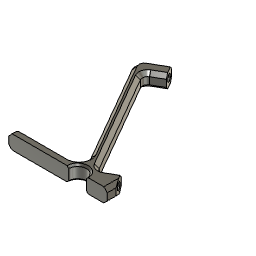
CYD Stand Leg Portrait (Autodesk Fusion 360 design; units mm, degrees)
Autodesk Fusion 360 part; units mm, degrees
sketch "Sketch1" plane through (0, 0, 0) normal (0, 0, 1) x (1, 0, 0)
  line L0 (0, 0) -> (55.9904, 0)
  line L1 (55.9904, 0) -> (55.9904, 5)
  line L2 (30.0096, 5) -> (3, 5)
  line L3 (0, 5) -> (0, 0)
  line L4 (34.3397, 12.5) -> (2.5, 67.6481)
  line L5 (41.5566, 0) -> (125.219, 0) construction
  line L6 (9.8301, 64.9519) -> (41.8301, 9.5263)
  line L7 (4.3301, 74.4782) -> (12.9904, 79.4782)
  line L8 (12.9904, 79.4782) -> (16.9904, 72.55)
  line L9 (16.9904, 72.55) -> (10.9282, 69.05)
  line L10 (14.9904, 76.0141) -> (36.6637, 88.5272) construction
  line L11 (0, 2) -> (0, 0) construction
  line L12 (55.9904, 5) -> (51.9904, 11.9282)
  line L13 (51.9904, 11.9282) -> (45.9282, 8.4282)
  arc A0 (4.3301, 74.4782) -> (2.5, 67.6481) centre (6.8301, 70.1481) ccw
  arc A1 (3, 5) -> (0, 2) centre (3, 2) ccw
  arc A2 (30.0096, 5) -> (34.3397, 12.5) centre (30.0096, 10) ccw
  arc A3 (41.8301, 9.5263) -> (45.9282, 8.4282) centre (44.4282, 11.0263) ccw
  arc A4 (10.9282, 69.05) -> (9.8301, 64.9519) centre (12.4282, 66.4519) ccw
  arc A5 (44.1423, 0) -> (34.1423, 0) centre (39.1423, 0) ccw
  line L14 (53.9904, 8.4641) -> (45.1077, 3.3357) construction
  point P0 (0, 71.9782)
  dimension "d1" = 5
  dimension "d2" = 120
  dimension "d3" = 5
  dimension "d4" = 8
  dimension "d8" = 8
  dimension "d9" = 5
  dimension "d10" = 3
  dimension "d11" = 5
  dimension "d12" = 3
  dimension "d13" = 3
  dimension "d24" = 5
  dimension "d30" = 10
  dimension "d31" = 5
  dimension "d32" = 78
  constraint horizontal L0
  constraint vertical L1
  constraint horizontal L2
  constraint coincident L0.start L3.end
  constraint horizontal L5
  constraint coincident L0 L5.start
  constraint perpendicular L7 L8
  constraint perpendicular L8 L9
  constraint midpoint L8 L10.start
  constraint perpendicular L8 L10
  constraint perpendicular L6 L9
  constraint coincident L0 L3.end
  constraint perpendicular L0 L11
  constraint collinear L3 L11
  constraint collinear L8 L12
  constraint perpendicular L6 L13
  constraint coincident P0 L4
  constraint tangent L4 A0
  constraint coincident L7.start A0.start
  constraint coincident P0 L11
  constraint coincident L3.start L2
  constraint tangent L11 A1
  constraint tangent L2 A1
  constraint coincident L1.end L2
  constraint coincident L5.start L4
  constraint tangent L2 A2
  constraint tangent L4 A2
  constraint tangent L6 A3
  constraint tangent L13 A3
  constraint coincident L7.start L6
  constraint tangent L9 A4
  constraint tangent L6 A4
  constraint coincident L0 A5.start
  constraint coincident L0 A5.centre
  constraint midpoint L12 L14.start
  constraint perpendicular L12 L14
  measures "d1" distance of L0.start L3.start
  measures "d2" angle of L4 L5
  measures "d3" distance of P0 L7.start
  measures "d4" distance of L7.end L8.end
  measures "d8" distance of L1.end L12.end
  measures "d9" radius of A0
  measures "d10" radius of A1
  measures "d11" radius of A2
  measures "d12" radius of A3
  measures "d13" radius of A4
  measures "d24" radius of A5
  measures "d30" distance of L6 L8
  measures "d31" distance of L4 L6
  measures "d32" distance of L10 L14
extrude "Extrude1" add sketch "Sketch1" along normal blind 8 contours L0 L1 L2 L3 L4 L6 L7 L8 L9 L12 L13 A0 A1 A2 A3 A4 A5
sketch "Sketch2" plane through (44.1578, 25.4945, 0) normal (0.866025, 0.5, 0) x (-0.5, 0.866025, 0)
  line L0 (54.3349, 0) -> (62.3349, 0)
  line L1 (62.3349, 0) -> (62.3349, 8)
  line L2 (62.3349, 8) -> (54.3349, 8)
  line L3 (54.3349, 8) -> (54.3349, 0)
  line L4 (-23.6651, 0) -> (-15.6651, 0) construction
  line L5 (-15.6651, 0) -> (-15.6651, 8) construction
  line L6 (-15.6651, 8) -> (-23.6651, 8) construction
  line L7 (-23.6651, 8) -> (-23.6651, 0) construction
  line L8 (54.3349, 8) -> (62.3349, 0) construction
  line L9 (62.3349, 8) -> (54.3349, 0) construction
  line L10 (-23.6651, 8) -> (-15.6651, 0) construction
  line L11 (-15.6651, 8) -> (-23.6651, 0) construction
  circle A0 centre (-19.6651, 4) radius 2
  circle A1 centre (58.3349, 4) radius 2
  circle A2 centre (-19.6651, 4) radius 1.6
  circle A3 centre (58.3349, 4) radius 1.6
  dimension "d16" = 4
  dimension "d17" = 4
  dimension "d26" = 3.2
  dimension "d27" = 3.2
  constraint coincident L2.end L3.start
  constraint coincident L0.end L1.start
  constraint coincident L1.end L2.start
  constraint coincident L0.start L3.end
  constraint coincident L6.end L7.start
  constraint coincident L4.end L5.start
  constraint coincident L5.end L6.start
  constraint coincident L4.start L7.end
  constraint midpoint L10 A0.centre
  constraint midpoint L8 A1.centre
  constraint concentric A0 A2
  constraint concentric A1 A3
  measures "d16" diameter of A0
  measures "d17" diameter of A1
  measures "d26" diameter of A2
  measures "d27" diameter of A3
extrude "Extrude2" cut sketch "Sketch2" against normal blind 4 contours A0 | A1 | A2 | A3
extrude "Extrude3" cut sketch "Sketch2" against normal blind 10 contours A2 | A3
chamfer "Chamfer1" distance 2 angle 45 26 edges at (16.5048, 5, 8) (34.3397, 7.5, 8) (18.4199, 40.074, 8) (2.0005, 71.4422, 8) (8.6602, 76.9782, 8) (0, 1, 8) (0.8787, 4.1213, 8) (25.8301, 37.2391, 8) (43.6517, 8.1285, 8) (48.9593, 10.1782, 8) (13.9593, 70.8, 8) (9.5304, 67.2284, 8) (25.8301, 37.2391, 0) (9.5304, 67.2284, 0) (13.9593, 70.8, 0) (48.9593, 10.1782, 0) (43.6517, 8.1285, 0) (18.4199, 40.074, 0) (34.3397, 7.5, 0) (16.5048, 5, 0) (0.8787, 4.1213, 0) (0, 1, 0) (8.6602, 76.9782, 0) (2.0005, 71.4422, 0) (55.9904, 2.5, 8) (55.9904, 2.5, 0)
chamfer "Chamfer2" distance 1 angle 45 2 edges at (39.1423, 5, 0) (39.1423, 5, 8)
named bodies: "Stand Leg Landscape"
